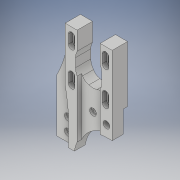
# Autodesk Inventor part: nema17-mount-right
Saved by Autodesk Inventor 2018 (Build 220112000, 112)
## iProperties
Created: 2017-10-08
Part Number: nema17-mount-right
Material: Generic
Document SubType Name: Modeling
Designer: Jurjen
Density: 1 g/cm^3
Appearance: Default
Author: Jurjen
Autodesk Inventor part; units mm, degrees
ref_plane "YZ Plane" through (0, 0, 0) normal (1, 0, 0) x (0, 1, 0)
sketch "Sketch1" plane through (0, 0, 0) normal (0, 0, 1) x (1, 0, 0)
  line L0 (21.5, 48.5) -> (21.5, -48.5)
  line L1 (21.5, -48.5) -> (-21.5, -48.5)
  line L2 (-21.5, -48.5) -> (-21.5, 48.5)
  line L3 (10.5, 48.5) -> (10.5, 6.5)
  line L4 (10.5, 6.5) -> (-10.5, 6.5)
  line L5 (-10.5, 6.5) -> (-10.5, 48.5)
  line L6 (-21.5, 48.5) -> (-10.5, 48.5)
  line L7 (10.5, 48.5) -> (21.5, 48.5)
  point P0 (0, 0)
  point P1 (21.5, 0)
  point P2 (0, -48.5)
  dimension "d0" = 97
  dimension "d1" = 43
  dimension "d2" = 11
  dimension "d3" = 11
  dimension "d4" = 42
  constraints: 16 end point, 4 parallel, 3 horizontal alignment, 2 horizontal, 2 midpoint, 2 perpendicular, 1 vertical alignment
  measures "d0" distance of L0.start L0.end
  measures "d1" distance between parallel lines of L0 L2
  measures "d2" distance between parallel lines of L2 L5
  measures "d3" distance between parallel lines of L0 L3
  measures "d4" distance between parallel lines of L7 L4
extrude "Extrusion1" add sketch "Sketch1" along normal mid plane 6
sketch "Sketch2" plane through (0, 0, 3) normal (0, 0, 1) x (1, 0, 0)
  arc A0 (-13.9, 41.5) -> (-17.1, 41.5) centre (-15.5, 41.5) ccw
  arc A1 (-13.9, 10.5) -> (-17.1, 10.5) centre (-15.5, 10.5) ccw
  arc A2 (17.1, 10.5) -> (13.9, 10.5) centre (15.5, 10.5) ccw
  arc A3 (17.1, 41.5) -> (13.9, 41.5) centre (15.5, 41.5) ccw
  line L0 (-15.5, 41.5) -> (15.5, 41.5) construction
  line L1 (10.5, 6.5) -> (-10.5, 6.5) projected
  line L2 (-10.5, 48.5) -> (-21.5, 48.5) projected
  arc A4 (-17.1, 33.5) -> (-13.9, 33.5) centre (-15.5, 33.5) ccw
  arc A5 (-17.1, 2.5) -> (-13.9, 2.5) centre (-15.5, 2.5) ccw
  arc A6 (13.9, 2.5) -> (17.1, 2.5) centre (15.5, 2.5) ccw
  arc A7 (13.9, 33.5) -> (17.1, 33.5) centre (15.5, 33.5) ccw
  line L3 (-17.1, 33.5) -> (-17.1, 41.5)
  line L4 (-13.9, 33.5) -> (-13.9, 41.5)
  line L5 (13.9, 33.5) -> (13.9, 41.5)
  line L6 (17.1, 33.5) -> (17.1, 41.5)
  line L7 (-17.1, 10.5) -> (-17.1, 2.5)
  line L8 (-13.9, 2.5) -> (-13.9, 10.5)
  line L9 (13.9, 10.5) -> (13.9, 2.5)
  line L10 (17.1, 10.5) -> (17.1, 2.5)
  point P0 (0, 0)
  point P1 (0, 41.5)
  point P2 (0, 6.5)
  dimension "d7" = 31
  dimension "d8" = 31
  dimension "d9" = 3.2
  dimension "d10" = 7
  dimension "d11" = 8
  dimension "d12" = 8
  constraints: 18 end point, 16 point on circle, 9 point on line, 8 centre point, 7 equal radius, 7 vertical alignment, 3 horizontal alignment, 3 tangent, 2 midpoint, 2 parallel, 1 horizontal, 1 vertical
  measures "d7" distance of L0.end L0.start
  measures "d8" distance of A1.centre L0.start
  measures "d9" diameter of A0
  measures "d10" distance from line of L2 L0.start
  measures "d11" distance of L3.start L3.end
  measures "d12" distance of L7.start L7.end
extrude "Extrusion2" cut sketch "Sketch2" against normal up to next
fillet "Fillet1" radius 8 2 edges at (10.5, 6.5, 0) (-10.5, 6.5, 0)
sketch "Sketch3" plane through (0, 0, 3) normal (0, 0, 1) x (1, 0, 0)
  line L0 (-17.1, 2.5) -> (-17.1, 10.5) projected
  arc A0 (-17.1, 2.5) -> (-13.9, 2.5) centre (-15.5, 2.5) ccw projected
  line L1 (-13.9, 10.5) -> (-13.9, 2.5) projected
  arc A1 (-13.9, 10.5) -> (-17.1, 10.5) centre (-15.5, 10.5) ccw projected
  line L2 (-13.9, 41.5) -> (-13.9, 33.5) projected
  arc A2 (-17.1, 33.5) -> (-13.9, 33.5) centre (-15.5, 33.5) ccw projected
  line L3 (-17.1, 33.5) -> (-17.1, 41.5) projected
  arc A3 (-13.9, 41.5) -> (-17.1, 41.5) centre (-15.5, 41.5) ccw projected
  line L4 (17.1, 10.5) -> (17.1, 2.5) projected
  arc A4 (13.9, 2.5) -> (17.1, 2.5) centre (15.5, 2.5) ccw projected
  line L5 (13.9, 2.5) -> (13.9, 10.5) projected
  arc A5 (17.1, 10.5) -> (13.9, 10.5) centre (15.5, 10.5) ccw projected
  line L6 (17.1, 41.5) -> (17.1, 33.5) projected
  arc A6 (13.9, 33.5) -> (17.1, 33.5) centre (15.5, 33.5) ccw projected
  line L7 (13.9, 33.5) -> (13.9, 41.5) projected
  arc A7 (17.1, 41.5) -> (13.9, 41.5) centre (15.5, 41.5) ccw projected
  line L8 (-17.1, 2.5) -> (-17.1, 10.5) projected
  arc A8 (-13.9, 10.5) -> (-17.1, 10.5) centre (-15.5, 10.5) ccw projected
  line L9 (-13.9, 10.5) -> (-13.9, 2.5) projected
  arc A9 (-17.1, 2.5) -> (-13.9, 2.5) centre (-15.5, 2.5) ccw projected
  line L10 (-13.9, 41.5) -> (-13.9, 33.5) projected
  arc A10 (-17.1, 33.5) -> (-13.9, 33.5) centre (-15.5, 33.5) ccw projected
  line L11 (-17.1, 33.5) -> (-17.1, 41.5) projected
  arc A11 (-13.9, 41.5) -> (-17.1, 41.5) centre (-15.5, 41.5) ccw projected
  line L12 (17.1, 41.5) -> (17.1, 33.5) projected
  arc A12 (13.9, 33.5) -> (17.1, 33.5) centre (15.5, 33.5) ccw projected
  line L13 (13.9, 33.5) -> (13.9, 41.5) projected
  arc A13 (17.1, 41.5) -> (13.9, 41.5) centre (15.5, 41.5) ccw projected
  line L14 (13.9, 2.5) -> (13.9, 10.5) projected
  arc A14 (17.1, 10.5) -> (13.9, 10.5) centre (15.5, 10.5) ccw projected
  line L15 (17.1, 10.5) -> (17.1, 2.5) projected
  arc A15 (13.9, 2.5) -> (17.1, 2.5) centre (15.5, 2.5) ccw projected
  line L16 (-21.5, 48.5) -> (-21.5, -48.5) projected
  line L17 (-21.5, -48.5) -> (21.5, -48.5) projected
  line L18 (21.5, -48.5) -> (21.5, 48.5) projected
  line L19 (21.5, 48.5) -> (10.5, 48.5) projected
  line L20 (10.5, 48.5) -> (10.5, 14.5) projected
  arc A16 (2.5, 6.5) -> (10.5, 14.5) centre (2.5, 14.5) ccw projected
  line L21 (2.5, 6.5) -> (-2.5, 6.5) projected
  arc A17 (-10.5, 14.5) -> (-2.5, 6.5) centre (-2.5, 14.5) ccw projected
  line L22 (-10.5, 14.5) -> (-10.5, 48.5) projected
  line L23 (-10.5, 48.5) -> (-21.5, 48.5) projected
  line L24 (-10.5, 14.5) -> (-10.5, 48.5) projected
  line L25 (-10.5, 48.5) -> (-10.5, -48.5)
  line L26 (21.5, -48.5) -> (-21.5, -48.5) projected
  line L27 (10.5, 48.5) -> (10.5, -48.5)
  point P0 (0, 0)
  constraints: 4 end point, 2 point on line, 1 perpendicular, 1 vertical
extrude "Extrusion3" add sketch "Sketch3" along normal blind 4 contours L23 L22 L25 L17 L16 | L27 L20 L19 L18 L17
sketch "Sketch4" plane through (0, 0, 7) normal (0, 0, 1) x (1, 0, 0)
  arc A0 (17.1, 10.5) -> (13.9, 10.5) centre (15.5, 10.5) ccw projected
  line L0 (13.9, 2.5) -> (13.9, 10.5) projected
  arc A1 (13.9, 2.5) -> (17.1, 2.5) centre (15.5, 2.5) ccw projected
  line L1 (17.1, 10.5) -> (17.1, 2.5) projected
  arc A2 (13.9, 33.5) -> (17.1, 33.5) centre (15.5, 33.5) ccw projected
  line L2 (13.9, 33.5) -> (13.9, 41.5) projected
  line L3 (17.1, 41.5) -> (17.1, 33.5) projected
  arc A3 (17.1, 41.5) -> (13.9, 41.5) centre (15.5, 41.5) ccw projected
  line L4 (-17.1, 2.5) -> (-17.1, 10.5) projected
  arc A4 (-17.1, 33.5) -> (-13.9, 33.5) centre (-15.5, 33.5) ccw projected
  line L5 (-17.1, 33.5) -> (-17.1, 41.5) projected
  arc A5 (-13.9, 41.5) -> (-17.1, 41.5) centre (-15.5, 41.5) ccw projected
  line L6 (-13.9, 41.5) -> (-13.9, 33.5) projected
  arc A6 (-13.9, 10.5) -> (-17.1, 10.5) centre (-15.5, 10.5) ccw projected
  line L7 (-13.9, 10.5) -> (-13.9, 2.5) projected
  arc A7 (-17.1, 2.5) -> (-13.9, 2.5) centre (-15.5, 2.5) ccw projected
  line L8 (-17.1, 2.5) -> (-17.1, 10.5) projected
  line L9 (-21.5, 48.5) -> (-21.5, -48.5) projected
  line L10 (-21.5, -48.5) -> (-10.5, -48.5) projected
  line L11 (-10.5, -48.5) -> (-10.5, 48.5) projected
  line L12 (-10.5, 48.5) -> (-21.5, 48.5) projected
  line L13 (-12.5, 2.5) -> (-12.5, 10.5)
  arc A8 (-12.5, 10.5) -> (-18.5, 10.5) centre (-15.5, 10.5) ccw
  line L14 (-18.5, 10.5) -> (-18.5, 2.5)
  arc A9 (-18.5, 2.5) -> (-12.5, 2.5) centre (-15.5, 2.5) ccw
  arc A10 (-18.5, 33.5) -> (-12.5, 33.5) centre (-15.5, 33.5) ccw
  line L15 (-18.5, 33.5) -> (-18.5, 41.5)
  arc A11 (-12.5, 41.5) -> (-18.5, 41.5) centre (-15.5, 41.5) ccw
  line L16 (-12.5, 41.5) -> (-12.5, 33.5)
  arc A12 (12.5, 2.5) -> (18.5, 2.5) centre (15.5, 2.5) ccw
  line L17 (12.5, 2.5) -> (12.5, 10.5)
  arc A13 (18.5, 10.5) -> (12.5, 10.5) centre (15.5, 10.5) ccw
  line L18 (18.5, 10.5) -> (18.5, 2.5)
  arc A14 (12.5, 33.5) -> (18.5, 33.5) centre (15.5, 33.5) ccw
  line L19 (12.5, 33.5) -> (12.5, 41.5)
  arc A15 (18.5, 41.5) -> (12.5, 41.5) centre (15.5, 41.5) ccw
  line L20 (18.5, 41.5) -> (18.5, 33.5)
  point P0 (0, 0)
  dimension "d18" = 6
  dimension "d20" = 6
  constraints: 16 end point, 16 point on circle, 8 centre point, 2 vertical alignment, 12 other
  measures "d18" distance between parallel lines of L17 L18
  measures "d20" distance between parallel lines of L14 L13
extrude "Extrusion4" cut sketch "Sketch4" against normal blind 4 contours A9 L14 A8 L13 | L15 A11 L16 A10 | L17 A13 L18 A12 | L19 A15 L20 A14
sketch "Sketch5" plane through (0, 0, 7) normal (0, 0, 1) x (1, 0, 0)
  arc A0 (-12, 18) -> (12, 18) centre (0, 18) ccw
  arc A1 (12, 26) -> (-12, 26) centre (0, 26) ccw
  line L0 (-17.1, 10.5) -> (-17.1, 2.5) projected
  arc A2 (-13.9, 10.5) -> (-17.1, 10.5) centre (-15.5, 10.5) ccw projected
  line L1 (-13.9, 2.5) -> (-13.9, 10.5) projected
  arc A3 (-17.1, 2.5) -> (-13.9, 2.5) centre (-15.5, 2.5) ccw projected
  line L2 (-12.5, 10.5) -> (-12.5, 2.5) projected
  arc A4 (-12.5, 10.5) -> (-18.5, 10.5) centre (-15.5, 10.5) ccw projected
  line L3 (-18.5, 2.5) -> (-18.5, 10.5) projected
  arc A5 (-18.5, 2.5) -> (-12.5, 2.5) centre (-15.5, 2.5) ccw projected
  line L4 (-12, 18) -> (-12, 26)
  line L5 (12, 18) -> (12, 26)
  point P0 (0, 0)
  dimension "d23" = 24
  dimension "d24" = 8
  dimension "d25" = 15.5
  constraints: 5 point on circle, 4 end point, 4 tangent, 2 centre point, 2 vertical alignment, 1 equal radius, 1 point on line, 1 vertical
  measures "d23" diameter of A0
  measures "d24" distance of A1.centre A0.centre
  measures "d25" horizontal distance of A0.centre A3.centre
extrude "Extrusion5" cut sketch "Sketch5" against normal up to surface (10 mm away) contours L4 A1 L5 A0
ref_plane "Work Plane1" through (-15.5, 2.5, -3) normal (1, 0, 0) x (0, 0, -1)
ref_plane "Work Plane2" through (15.5, 2.5, -3) normal (1, 0, 0) x (0, 0, -1)
sketch "Sketch10" plane through (0, 0, -3) normal (0, 0, -1) x (-1, 0, 0)
  line L0 (-13.9, 10.5) -> (-13.9, 2.5) projected
  arc A0 (-17.1, 2.5) -> (-13.9, 2.5) centre (-15.5, 2.5) ccw projected
  line L1 (-17.1, 2.5) -> (-17.1, 10.5) projected
  arc A1 (-13.9, 10.5) -> (-17.1, 10.5) centre (-15.5, 10.5) ccw projected
  line L2 (-17.1, 33.5) -> (-17.1, 41.5) projected
  arc A2 (-13.9, 41.5) -> (-17.1, 41.5) centre (-15.5, 41.5) ccw projected
  line L3 (-13.9, 41.5) -> (-13.9, 33.5) projected
  arc A3 (-17.1, 33.5) -> (-13.9, 33.5) centre (-15.5, 33.5) ccw projected
  line L4 (13.9, 33.5) -> (13.9, 41.5) projected
  arc A4 (17.1, 41.5) -> (13.9, 41.5) centre (15.5, 41.5) ccw projected
  line L5 (17.1, 41.5) -> (17.1, 33.5) projected
  arc A5 (13.9, 33.5) -> (17.1, 33.5) centre (15.5, 33.5) ccw projected
  line L6 (17.1, 10.5) -> (17.1, 2.5) projected
  arc A6 (13.9, 2.5) -> (17.1, 2.5) centre (15.5, 2.5) ccw projected
  line L7 (13.9, 2.5) -> (13.9, 10.5) projected
  arc A7 (17.1, 10.5) -> (13.9, 10.5) centre (15.5, 10.5) ccw projected
  arc A8 (12, 26) -> (10.5, 31.8095) centre (0, 26) ccw projected
  line L8 (12, 26) -> (12, 18) projected
  arc A9 (9.5768, 10.7691) -> (12, 18) centre (0, 18) ccw projected
  arc A10 (3.7341, 6.5958) -> (9.5768, 10.7691) centre (2.5, 14.5) ccw projected
  arc A11 (-3.7341, 6.5958) -> (3.7341, 6.5958) centre (0, 18) ccw projected
  arc A12 (-9.5768, 10.7691) -> (-3.7341, 6.5958) centre (-2.5, 14.5) ccw projected
  line L9 (-12, 18) -> (-12, 26) projected
  arc A13 (-10.5, 31.8095) -> (-12, 26) centre (0, 26) ccw projected
  line L10 (-10.5, 31.8095) -> (-10.5, 48.5) projected
  line L11 (-10.5, 48.5) -> (-21.5, 48.5) projected
  line L12 (-21.5, -48.5) -> (21.5, -48.5) projected
  line L13 (21.5, -48.5) -> (21.5, 48.5) projected
  line L14 (21.5, 48.5) -> (10.5, 48.5) projected
  line L15 (10.5, 48.5) -> (10.5, 31.8095) projected
  line L16 (15.5, 2.5) -> (15.5, -3) construction
  circle A14 centre (0, -13) radius 2.1
  circle A15 centre (-16.3, -13) radius 2.1
  line L17 (10.5, -48.5) -> (-10.5, -48.5) projected
  arc A16 (-12, 18) -> (-9.5768, 10.7691) centre (0, 18) ccw projected
  line L18 (-21.5, 48.5) -> (-21.5, -48.5) projected
  point P0 (0, 0)
  point P1 (0, -48.5)
  dimension "d43" = 5.5
  dimension "d44" = 4.2
  dimension "d47" = 10
  dimension "d78" = 5.2
  constraints: 2 centre point, 2 end point, 1 equal radius, 1 horizontal alignment, 1 midpoint, 1 vertical, 1 vertical alignment
  measures "d43" distance of L16.start L16.end
  measures "d44" diameter of A15
  measures "d47" vertical distance of A15.centre L16.end
  measures "d78" distance from line of L18 A15.centre
extrude "Extrusion9" cut sketch "Sketch10" against normal up to next contours A14 | A15
sketch "Sketch12" plane through (0, 0, 7) normal (0, 0, 1) x (1, 0, 0)
  circle A0 centre (16.3, -13) radius 2.1 projected
  circle A1 centre (16.3, -13) radius 3.1
  circle A2 centre (0, -13) radius 2.1 projected
  circle A3 centre (0, -13) radius 3.1
  point P0 (0, 0)
  dimension "d79" = 6.2
  constraints: 2 centre point, 1 coincident, 1 equal radius
  measures "d79" diameter of A1
sketch "Sketch14" plane through (0, 0, -3) normal (0, 0, -1) x (-1, 0, 0)
  line L0 (0, 26) -> (33, 26) construction
  line L1 (21.5, -48.5) -> (21.5, 48.5) construction
  arc A0 (21.5, 48.5) -> (33, 0) centre (129.72, 48.547) ccw
  line L2 (33, 0) -> (33, -48.5)
  line L3 (33, -48.5) -> (21.5, -48.5)
  line L4 (21.5, 48.5) -> (21.5, -48.5)
  point P0 (0, 0)
  point P1 (12, 26)
  dimension "d69" = 33
  dimension "d70" = 108.22
  constraints: 8 end point, 2 perpendicular, 2 point on circle, 2 vertical alignment, 1 centre point, 1 horizontal, 1 horizontal alignment, 1 vertical
  measures "d69" distance of L0.start L0.end
  measures "d70" radius of A0
extrude "Extrusion13" add sketch "Sketch14" against normal up to surface (6 mm away)
sketch "Sketch15" plane through (0, 0, 7) normal (0, 0, 1) x (1, 0, 0)
  line L0 (-21.5, 48.5) -> (-21.5, -48.5) projected
  arc A0 (-18.5, -21.5) -> (-21.5, 0) centre (-197.9485, -35.58) ccw
  line L1 (-18.5, -21.5) -> (-18.5, -48.5)
  line L2 (-18.5, -48.5) -> (-21.5, -48.5)
  line L3 (-21.5, 0) -> (-21.5, -48.5)
  point P0 (0, 0)
  dimension "d73" = 3
  dimension "d74" = 27
  dimension "d75" = 180
  constraints: 6 end point, 2 point on circle, 1 centre point, 1 collinear, 1 midpoint, 1 perpendicular, 1 vertical
  measures "d73" distance between parallel lines of L0 L1
  measures "d74" distance of L1.start L1.end
  measures "d75" radius of A0
extrude "Extrusion14" cut sketch "Sketch15" against normal up to surface (4 mm away)
extrude "Extrusion15" cut sketch "Sketch12" against normal blind 6
sketch "Sketch16" plane through (-33, -48.5, 3) normal (0, 0, 1) x (1, 0, 0)
  circle A0 centre (10, 8) radius 2.1
  line L0 (0, 0) -> (0, 48.5) projected
  circle A1 centre (10, 20) radius 2.1
  line L1 (14.5, 0) -> (0, 0) projected
  point P0 (33, 48.5)
  dimension "d82" = 10
  dimension "d83" = 4.2
  dimension "d84" = 4.2
  dimension "d85" = 8
  dimension "d86" = 12
  constraints: 2 centre point, 1 vertical alignment
  measures "d82" distance from line of L0 A0.centre
  measures "d83" diameter of A0
  measures "d84" diameter of A1
  measures "d85" distance from line of L1 A0.centre
  measures "d86" distance of A0.centre A1.centre
extrude "Extrusion16" cut sketch "Sketch16" against normal up to next
sketch "Sketch17" plane through (-33, -48.5, 3) normal (0, 0, 1) x (1, 0, 0)
  circle A0 centre (10, 8) radius 2.1 projected
  circle A1 centre (10, 20) radius 2.1 projected
  circle A2 centre (10, 8) radius 3.1
  circle A3 centre (10, 20) radius 3.1
  point P0 (33, 48.5)
  dimension "d89" = 6.2
  constraints: 2 centre point, 1 equal radius
  measures "d89" diameter of A2
extrude "Extrusion17" cut sketch "Sketch17" against normal blind 2
sketch "Sketch18" plane through (0, 0, -3) normal (0, 0, -1) x (-1, 0, 0)
  line L0 (18.5, -48.5) -> (33, -48.5) projected
  line L1 (33, -48.5) -> (13, -48.5)
  circle A0 centre (-16.3, -13) radius 2.1 projected
  line L2 (-16.3, -13) -> (-16.3, -23) construction
  arc A1 (13, -48.5) -> (-16.3, -23) centre (-16.3, -52.5831) ccw
  line L3 (-16.3, -23) -> (-21.5, -23)
  line L4 (-21.5, 48.5) -> (-21.5, -48.5) projected
  line L5 (-21.5, -48.5) -> (13, -48.5)
  line L6 (-21.5, -48.5) -> (33, -48.5) projected
  line L7 (-21.5, -48.5) -> (-21.5, -23)
  point P0 (0, 0)
  dimension "d93" = 20
  dimension "d94" = 10
  constraints: 10 end point, 2 collinear, 2 point on circle, 1 centre point, 1 horizontal, 1 line through centre, 1 perpendicular, 1 point on line, 1 vertical
  measures "d93" distance of L0.end L1.end
  measures "d94" distance of L2.start L2.end
extrude "Extrusion18" cut sketch "Sketch18" against normal up to next contours L5 L4 L3 A1
sketch "Sketch19" plane through (0, 0, -3) normal (0, 0, -1) x (-1, 0, 0)
  line L0 (-21.5, -23) -> (-21.5, 48.5) projected
  line L1 (-21.5, -3) -> (33, -3)
  line L2 (33, -48.5) -> (33, 0) construction
  circle A0 centre (-16.3, -13) radius 2.1 construction
  line L3 (-16.3, -13) -> (-16.3, -3) construction
  line L4 (-21.5, -23) -> (-16.3, -23) construction
  arc A1 (13, -48.5) -> (-16.3, -23) centre (-16.3, -52.5831) ccw construction
  line L5 (13, -48.5) -> (33, -48.5) construction
  line L6 (33, -48.5) -> (33, 0) projected
  arc A2 (21.5, 48.5) -> (33, 0) centre (129.72, 48.547) ccw projected
  line L7 (21.5, 48.5) -> (10.5, 48.5) projected
  line L8 (10.5, 48.5) -> (10.5, 31.8095) projected
  arc A3 (12, 26) -> (10.5, 31.8095) centre (0, 26) ccw projected
  line L9 (12, 26) -> (12, 18) projected
  arc A4 (9.5768, 10.7691) -> (12, 18) centre (0, 18) ccw projected
  arc A5 (3.7341, 6.5958) -> (9.5768, 10.7691) centre (2.5, 14.5) ccw projected
  arc A6 (-3.7341, 6.5958) -> (3.7341, 6.5958) centre (0, 18) ccw projected
  arc A7 (-9.5768, 10.7691) -> (-3.7341, 6.5958) centre (-2.5, 14.5) ccw projected
  arc A8 (-12, 18) -> (-9.5768, 10.7691) centre (0, 18) ccw projected
  line L10 (-12, 18) -> (-12, 26) projected
  arc A9 (-10.5, 31.8095) -> (-12, 26) centre (0, 26) ccw projected
  line L11 (-10.5, 31.8095) -> (-10.5, 48.5) projected
  line L12 (-10.5, 48.5) -> (-21.5, 48.5) projected
  line L13 (-21.5, 48.5) -> (-21.5, -23) projected
  line L14 (17.1, 10.5) -> (17.1, 2.5) projected
  arc A10 (13.9, 2.5) -> (17.1, 2.5) centre (15.5, 2.5) ccw projected
  line L15 (13.9, 2.5) -> (13.9, 10.5) projected
  arc A11 (17.1, 10.5) -> (13.9, 10.5) centre (15.5, 10.5) ccw projected
  line L16 (13.9, 33.5) -> (13.9, 41.5) projected
  arc A12 (17.1, 41.5) -> (13.9, 41.5) centre (15.5, 41.5) ccw projected
  line L17 (17.1, 41.5) -> (17.1, 33.5) projected
  arc A13 (13.9, 33.5) -> (17.1, 33.5) centre (15.5, 33.5) ccw projected
  line L18 (-17.1, 33.5) -> (-17.1, 41.5) projected
  arc A14 (-13.9, 41.5) -> (-17.1, 41.5) centre (-15.5, 41.5) ccw projected
  line L19 (-13.9, 41.5) -> (-13.9, 33.5) projected
  arc A15 (-17.1, 33.5) -> (-13.9, 33.5) centre (-15.5, 33.5) ccw projected
  line L20 (-13.9, 10.5) -> (-13.9, 2.5) projected
  arc A16 (-17.1, 2.5) -> (-13.9, 2.5) centre (-15.5, 2.5) ccw projected
  line L21 (-17.1, 2.5) -> (-17.1, 10.5) projected
  arc A17 (-13.9, 10.5) -> (-17.1, 10.5) centre (-15.5, 10.5) ccw projected
  circle A18 centre (-16.3, -13) radius 2.1 projected
  circle A19 centre (0, -13) radius 2.1 construction
  circle A20 centre (23, -28.5) radius 2.1 construction
  circle A21 centre (23, -40.5) radius 2.1 projected
  line L22 (33, -3) -> (33, 0)
  line L23 (-10.5, 48.5) -> (-21.5, 48.5) projected
  line L24 (-21.5, -3) -> (-21.5, 48.5)
  line L25 (-21.5, 48.5) -> (-21.5, -23) projected
  line L26 (-21.5, 48.5) -> (-10.5, 48.5)
  line L27 (-10.5, 31.8095) -> (-10.5, 48.5) projected
  line L28 (-10.5, 31.8095) -> (-10.5, 48.5)
  point P0 (0, 0)
  dimension "d97" = 10
  constraints: 12 end point, 3 perpendicular, 3 point on line, 1 collinear, 1 horizontal, 1 vertical
  measures "d97" distance of L3.start L3.end
extrude "Extrusion19" add sketch "Sketch19" along normal blind 4 contours L0 L12 L11 A9 L10 A8 A7 A6 A5 A4 L9 A3 L8 L7 A2 L6 L1
equation "\"d12\" = d11"
equation "\"d20\" = d18"
body "Solid1"
